Autodesk Fusion 360 part; units mm, degrees
(part 4 of 5)
  spline S979 degree 3 poles (-60.6177, -130.3554) (-60.6177, -130.0705) (-60.5544, -129.9545) (-60.3222, -129.8384) knots 0 0 0 0 1 1 1 1
  spline S980 degree 3 poles (-60.3222, -129.8384) (-60.1639, -129.754) (-60.0268, -129.6801) (-60.0162, -129.6695) knots 0 0 0 0 1 1 1 1
  spline S981 degree 2 poles (-60.0162, -129.6695) (-60.0795, -129.8911) (-60.1639, -130.1655) knots 0 0 0 1 1 1
  spline S982 degree 3 poles (-57.3993, -130.2816) (-56.819, -130.5665) (-56.1331, -130.9463) (-55.8798, -131.1152) knots 0 0 0 0 1 1 1 1
  line L170 (-55.8798, -131.1152) -> (-55.405, -131.4423)
  line L171 (-55.405, -131.4423) -> (-54.7508, -131.0308)
  spline S983 degree 3 poles (-54.7508, -131.0308) (-53.9805, -130.5665) (-53.0097, -130.06) (-52.9675, -130.1127) knots 0 0 0 0 1 1 1 1
  spline S984 degree 3 poles (-52.9675, -130.1127) (-52.9464, -130.1338) (-52.883, -130.5137) (-52.8197, -130.9674) knots 0 0 0 0 1 1 1 1
  spline S985 degree 3 poles (-52.8197, -130.9674) (-52.6931, -131.8855) (-52.672, -132.8985) (-52.767, -133.4894) knots 0 0 0 0 1 1 1 1
  line L172 (-52.767, -133.4894) -> (-52.8408, -133.8904)
  line L173 (-52.8408, -133.8904) -> (-53.379, -133.8904)
  spline S986 degree 3 poles (-53.379, -133.8904) (-53.9805, -133.8904) (-55.3733, -133.5527) (-55.616, -133.3522) knots 0 0 0 0 1 1 1 1
  spline S987 degree 3 poles (-55.616, -133.3522) (-55.9009, -133.1201) (-55.8693, -133.3206) (-55.5527, -133.6899) knots 0 0 0 0 1 1 1 1
  spline S988 degree 3 poles (-55.5527, -133.6899) (-55.3839, -133.8904) (-55.2467, -133.9959) (-55.2361, -133.9326) knots 0 0 0 0 1 1 1 1
  spline S989 degree 3 poles (-55.2361, -133.9326) (-55.2361, -133.8798) (-55.2995, -133.7637) (-55.3628, -133.6899) knots 0 0 0 0 1 1 1 1
  spline S990 degree 3 poles (-55.3628, -133.6899) (-55.4683, -133.5738) (-55.4683, -133.5632) (-55.3733, -133.616) knots 0 0 0 0 1 1 1 1
  spline S991 degree 3 poles (-55.3733, -133.616) (-55.2995, -133.6582) (-55.1517, -133.711) (-55.0568, -133.7321) knots 0 0 0 0 1 1 1 1
  spline S992 degree 3 poles (-55.0568, -133.7321) (-54.9512, -133.7532) (-54.5081, -133.8482) (-54.0754, -133.9431) knots 0 0 0 0 1 1 1 1
  spline S993 degree 3 poles (-54.0754, -133.9431) (-53.6428, -134.0381) (-53.2102, -134.1225) (-53.1152, -134.1331) knots 0 0 0 0 1 1 1 1
  spline S994 degree 3 poles (-53.1152, -134.1331) (-52.9675, -134.1436) (-52.9569, -134.1858) (-53.0835, -134.4918) knots 0 0 0 0 1 1 1 1
  spline S995 degree 3 poles (-53.0835, -134.4918) (-53.1679, -134.6818) (-53.2313, -134.9456) (-53.2313, -135.0827) knots 0 0 0 0 1 1 1 1
  spline S996 degree 3 poles (-53.2313, -135.0827) (-53.2313, -135.5576) (-53.3579, -135.5787) (-56.1225, -135.5681) knots 0 0 0 0 1 1 1 1
  spline S997 degree 3 poles (-56.1225, -135.5681) (-59.0243, -135.547) (-58.866, -135.5892) (-58.9188, -134.7978) knots 0 0 0 0 1 1 1 1
  spline S998 degree 3 poles (-58.9188, -134.7978) (-58.9399, -134.5657) (-59.0243, -134.2702) (-59.1087, -134.1331) knots 0 0 0 0 1 1 1 1
  spline S999 degree 3 poles (-59.1087, -134.1331) (-59.2565, -133.9115) (-59.2565, -133.8904) (-59.0771, -133.8904) knots 0 0 0 0 1 1 1 1
  spline S1000 degree 3 poles (-59.0771, -133.8904) (-58.961, -133.8904) (-58.6339, -133.9642) (-58.349, -134.0486) knots 0 0 0 0 1 1 1 1
  spline S1001 degree 3 poles (-58.349, -134.0486) (-57.8214, -134.2069) (-56.7451, -134.1858) (-56.2386, -133.9959) knots 0 0 0 0 1 1 1 1
  spline S1002 degree 3 poles (-56.2386, -133.9959) (-56.1225, -133.9537) (-55.8693, -133.9853) (-55.6582, -134.0697) knots 0 0 0 0 1 1 1 1
  line L174 (-55.6582, -134.0697) -> (-55.2889, -134.2175)
  line L175 (-55.2889, -134.2175) -> (-55.5527, -133.9959)
  spline S1003 degree 3 poles (-55.5527, -133.9959) (-55.7532, -133.8376) (-55.9009, -133.7954) (-56.1331, -133.8482) knots 0 0 0 0 1 1 1 1
  spline S1004 degree 3 poles (-56.1331, -133.8482) (-57.2621, -134.1014) (-58.6339, -134.0064) (-59.2143, -133.6266) knots 0 0 0 0 1 1 1 1
  spline S1005 degree 3 poles (-59.2143, -133.6266) (-59.6469, -133.3417) (-59.6469, -131.4845) (-59.2248, -130.0916) knots 0 0 0 0 1 1 1 1
  spline S1006 degree 3 poles (-59.2248, -130.0916) (-59.0982, -129.6801) (-59.0665, -129.659) (-58.7711, -129.7118) knots 0 0 0 0 1 1 1 1
  spline S1007 degree 3 poles (-58.7711, -129.7118) (-58.5917, -129.7434) (-57.9797, -130.0072) (-57.3993, -130.2816) knots 0 0 0 0 1 1 1 1
  spline S1008 degree 3 poles (-42.0883, -129.7434) (-42.1938, -129.8489) (-42.5737, -129.8595) (-42.5104, -129.754) knots 0 0 0 0 1 1 1 1
  spline S1009 degree 3 poles (-42.5104, -129.754) (-42.4787, -129.7118) (-42.3521, -129.6695) (-42.236, -129.6695) knots 0 0 0 0 1 1 1 1
  spline S1010 degree 3 poles (-42.236, -129.6695) (-42.1094, -129.6695) (-42.0461, -129.7012) (-42.0883, -129.7434) knots 0 0 0 0 1 1 1 1
  spline S1011 degree 3 poles (-48.7678, -132.3076) (-48.7572, -132.6241) (-48.7889, -132.9829) (-48.8205, -133.099) knots 0 0 0 0 1 1 1 1
  spline S1012 degree 3 poles (-48.8205, -133.099) (-48.9577, -133.5527) (-49.1054, -133.8693) (-49.2004, -133.9326) knots 0 0 0 0 1 1 1 1
  spline S1013 degree 3 poles (-49.2004, -133.9326) (-49.3587, -134.0275) (-49.2215, -133.5527) (-49.021, -133.3206) knots 0 0 0 0 1 1 1 1
  spline S1014 degree 3 poles (-49.021, -133.3206) (-48.8627, -133.1306) (-48.8627, -133.1201) (-49.0527, -133.1939) knots 0 0 0 0 1 1 1 1
  spline S1015 degree 3 poles (-49.0527, -133.1939) (-49.232, -133.2572) (-49.2426, -133.2256) (-49.1687, -132.8668) knots 0 0 0 0 1 1 1 1
  spline S1016 degree 3 poles (-49.1687, -132.8668) (-49.1371, -132.6452) (-49.0949, -132.3814) (-49.1054, -132.2759) knots 0 0 0 0 1 1 1 1
  spline S1017 degree 3 poles (-49.1054, -132.2759) (-49.1054, -132.1809) (-49.0632, -132.1176) (-49.021, -132.1493) knots 0 0 0 0 1 1 1 1
  spline S1018 degree 3 poles (-49.021, -132.1493) (-48.9682, -132.1704) (-48.9682, -131.991) (-49.021, -131.7483) knots 0 0 0 0 1 1 1 1
  spline S1019 degree 3 poles (-49.021, -131.7483) (-49.1476, -131.0835) (-49.116, -130.9463) (-48.9366, -131.3579) knots 0 0 0 0 1 1 1 1
  spline S1020 degree 3 poles (-48.9366, -131.3579) (-48.8522, -131.5584) (-48.7678, -131.991) (-48.7678, -132.3076) knots 0 0 0 0 1 1 1 1
  spline S1021 degree 3 poles (-50.2767, -134.1436) (-50.2767, -134.2175) (-50.3611, -134.4707) (-50.4561, -134.6923) knots 0 0 0 0 1 1 1 1
  spline S1022 degree 3 poles (-50.4561, -134.6923) (-50.551, -134.9245) (-50.6249, -135.1672) (-50.6038, -135.2516) knots 0 0 0 0 1 1 1 1
  spline S1023 degree 3 poles (-50.6038, -135.2516) (-50.5721, -135.4099) (-50.8043, -135.5892) (-50.9309, -135.5154) knots 0 0 0 0 1 1 1 1
  spline S1024 degree 3 poles (-50.9309, -135.5154) (-50.9731, -135.4837) (-51.0153, -135.3676) (-51.0153, -135.2516) knots 0 0 0 0 1 1 1 1
  spline S1025 degree 3 poles (-51.0153, -135.2516) (-51.0153, -135.1249) (-50.9731, -135.0722) (-50.8993, -135.1144) knots 0 0 0 0 1 1 1 1
  spline S1026 degree 3 poles (-50.8993, -135.1144) (-50.8148, -135.1672) (-50.8043, -135.1355) (-50.8782, -134.9983) knots 0 0 0 0 1 1 1 1
  spline S1027 degree 3 poles (-50.8782, -134.9983) (-51.0048, -134.7873) (-50.9415, -134.418) (-50.7832, -134.418) knots 0 0 0 0 1 1 1 1
  spline S1028 degree 3 poles (-50.7832, -134.418) (-50.7304, -134.418) (-50.7199, -134.3652) (-50.7621, -134.3019) knots 0 0 0 0 1 1 1 1
  spline S1029 degree 3 poles (-50.7621, -134.3019) (-50.836, -134.1753) (-50.6355, -133.9959) (-50.4033, -133.9959) knots 0 0 0 0 1 1 1 1
  spline S1030 degree 3 poles (-50.4033, -133.9959) (-50.34, -133.9959) (-50.2767, -134.0592) (-50.2767, -134.1436) knots 0 0 0 0 1 1 1 1
  spline S1031 degree 3 poles (-51.7645, -134.418) (-51.8173, -134.5868) (-51.9017, -134.8717) (-51.9545, -135.0405) knots 0 0 0 0 1 1 1 1
  spline S1032 degree 3 poles (-51.9545, -135.0405) (-52.0072, -135.2094) (-52.0178, -135.3887) (-51.9861, -135.431) knots 0 0 0 0 1 1 1 1
  spline S1033 degree 3 poles (-51.9861, -135.431) (-51.9439, -135.4732) (-51.9861, -135.4837) (-52.0705, -135.4521) knots 0 0 0 0 1 1 1 1
  spline S1034 degree 3 poles (-52.0705, -135.4521) (-52.2499, -135.3993) (-52.3238, -134.5235) (-52.1444, -134.5235) knots 0 0 0 0 1 1 1 1
  spline S1035 degree 3 poles (-52.1444, -134.5235) (-52.0811, -134.5235) (-52.0705, -134.4918) (-52.1022, -134.4496) knots 0 0 0 0 1 1 1 1
  spline S1036 degree 3 poles (-52.1022, -134.4496) (-52.1972, -134.3652) (-51.9756, -134.1014) (-51.7962, -134.1014) knots 0 0 0 0 1 1 1 1
  spline S1037 degree 3 poles (-51.7962, -134.1014) (-51.7012, -134.1014) (-51.6907, -134.1753) (-51.7645, -134.418) knots 0 0 0 0 1 1 1 1
  spline S1038 degree 3 poles (-53.2313, -111.3723) (-53.2313, -111.4462) (-53.1363, -111.6045) (-53.0097, -111.7417) knots 0 0 0 0 1 1 1 1
  spline S1039 degree 3 poles (-53.0097, -111.7417) (-52.8408, -111.9421) (-52.8197, -111.9527) (-52.9041, -111.7839) knots 0 0 0 0 1 1 1 1
  spline S1040 degree 3 poles (-52.9041, -111.7839) (-53.0835, -111.4251) (-53.2313, -111.2457) (-53.2313, -111.3723) knots 0 0 0 0 1 1 1 1
  spline S1041 degree 3 poles (-60.2378, -111.6889) (-60.3433, -111.8366) (-60.4066, -111.9843) (-60.375, -112.0055) knots 0 0 0 0 1 1 1 1
  spline S1042 degree 3 poles (-60.375, -112.0055) (-60.3539, -112.0371) (-60.2484, -111.9316) (-60.1534, -111.7733) knots 0 0 0 0 1 1 1 1
  spline S1043 degree 3 poles (-60.1534, -111.7733) (-60.0479, -111.6256) (-59.9846, -111.4779) (-60.0162, -111.4567) knots 0 0 0 0 1 1 1 1
  spline S1044 degree 3 poles (-60.0162, -111.4567) (-60.0373, -111.4251) (-60.1428, -111.5306) (-60.2378, -111.6889) knots 0 0 0 0 1 1 1 1
  spline S1045 degree 3 poles (-60.3433, -115.6248) (-60.3961, -115.7092) (-60.185, -115.7409) (-59.6152, -115.7409) knots 0 0 0 0 1 1 1 1
  spline S1046 degree 3 poles (-59.6152, -115.7409) (-59.1721, -115.7409) (-58.7183, -115.7936) (-58.6128, -115.8464) knots 0 0 0 0 1 1 1 1
  spline S1047 degree 3 poles (-58.6128, -115.8464) (-58.4018, -115.9625) (-58.2118, -115.8042) (-58.4123, -115.6881) knots 0 0 0 0 1 1 1 1
  spline S1048 degree 3 poles (-58.4123, -115.6881) (-58.6339, -115.5509) (-60.2695, -115.4982) (-60.3433, -115.6248) knots 0 0 0 0 1 1 1 1
  spline S1049 degree 3 poles (-52.4082, -116.9227) (-52.3554, -116.9755) (-52.2394, -117.0071) (-52.1655, -116.986) knots 0 0 0 0 1 1 1 1
  spline S1050 degree 3 poles (-52.1655, -116.986) (-52.0811, -116.9544) (-52.1338, -116.9121) (-52.271, -116.8699) knots 0 0 0 0 1 1 1 1
  spline S1051 degree 3 poles (-52.271, -116.8699) (-52.4504, -116.8277) (-52.4926, -116.8383) (-52.4082, -116.9227) knots 0 0 0 0 1 1 1 1
  spline S1052 degree 3 poles (-53.1785, -117.2182) (-53.2102, -117.2709) (-53.1996, -117.3237) (-53.1363, -117.3237) knots 0 0 0 0 1 1 1 1
  spline S1053 degree 3 poles (-53.1363, -117.3237) (-53.0835, -117.3237) (-52.9991, -117.2709) (-52.9675, -117.2182) knots 0 0 0 0 1 1 1 1
  spline S1054 degree 3 poles (-52.9675, -117.2182) (-52.9358, -117.1548) (-52.9464, -117.1126) (-53.0097, -117.1126) knots 0 0 0 0 1 1 1 1
  spline S1055 degree 3 poles (-53.0097, -117.1126) (-53.0624, -117.1126) (-53.1468, -117.1548) (-53.1785, -117.2182) knots 0 0 0 0 1 1 1 1
  spline S1056 degree 3 poles (-50.6249, -117.6086) (-50.6671, -117.6402) (-50.551, -117.7669) (-50.3822, -117.8724) knots 0 0 0 0 1 1 1 1
  spline S1057 degree 3 poles (-50.3822, -117.8724) (-49.9707, -118.1151) (-49.8441, -118.1151) (-50.1395, -117.8618) knots 0 0 0 0 1 1 1 1
  spline S1058 degree 3 poles (-50.1395, -117.8618) (-50.2661, -117.7563) (-50.34, -117.6402) (-50.3083, -117.598) knots 0 0 0 0 1 1 1 1
  spline S1059 degree 3 poles (-50.3083, -117.598) (-50.2661, -117.5664) (-50.3083, -117.5347) (-50.4033, -117.5347) knots 0 0 0 0 1 1 1 1
  spline S1060 degree 3 poles (-50.4033, -117.5347) (-50.4877, -117.5347) (-50.5933, -117.5664) (-50.6249, -117.6086) knots 0 0 0 0 1 1 1 1
  spline S1061 degree 3 poles (-61.8839, -117.9568) (-62.0105, -118.0412) (-62.0105, -118.0623) (-61.8312, -118.0623) knots 0 0 0 0 1 1 1 1
  spline S1062 degree 3 poles (-61.8312, -118.0623) (-61.7151, -118.0623) (-61.5463, -118.0096) (-61.4618, -117.9568) knots 0 0 0 0 1 1 1 1
  spline S1063 degree 3 poles (-61.4618, -117.9568) (-61.3352, -117.8724) (-61.3352, -117.8513) (-61.5146, -117.8513) knots 0 0 0 0 1 1 1 1
  spline S1064 degree 3 poles (-61.5146, -117.8513) (-61.6307, -117.8513) (-61.7995, -117.904) (-61.8839, -117.9568) knots 0 0 0 0 1 1 1 1
  spline S1065 degree 3 poles (-61.2086, -118.0307) (-61.1769, -118.094) (-61.2297, -118.1784) (-61.3141, -118.21) knots 0 0 0 0 1 1 1 1
  spline S1066 degree 3 poles (-61.3141, -118.21) (-61.3985, -118.2417) (-61.4618, -118.3261) (-61.4618, -118.3894) knots 0 0 0 0 1 1 1 1
  spline S1067 degree 3 poles (-61.4618, -118.3894) (-61.4618, -118.4633) (-61.3563, -118.4211) (-61.2191, -118.2945) knots 0 0 0 0 1 1 1 1
  spline S1068 degree 3 poles (-61.2191, -118.2945) (-61.082, -118.1678) (-60.8393, -118.0518) (-60.6599, -118.0518) knots 0 0 0 0 1 1 1 1
  spline S1069 degree 3 poles (-60.6599, -118.0518) (-60.4911, -118.0412) (-60.2062, -117.999) (-60.0373, -117.9568) knots 0 0 0 0 1 1 1 1
  spline S1070 degree 3 poles (-60.0373, -117.9568) (-59.8157, -117.904) (-59.9529, -117.8829) (-60.4805, -117.8935) knots 0 0 0 0 1 1 1 1
  spline S1071 degree 3 poles (-60.4805, -117.8935) (-61.0187, -117.904) (-61.2403, -117.9462) (-61.2086, -118.0307) knots 0 0 0 0 1 1 1 1
  spline S1072 degree 3 poles (-51.965, -118.8748) (-52.1022, -119.2652) (-52.2288, -119.6662) (-52.2605, -119.7506) knots 0 0 0 0 1 1 1 1
  spline S1073 degree 3 poles (-52.2605, -119.7506) (-52.2921, -119.8562) (-52.2816, -119.8773) (-52.1972, -119.8034) knots 0 0 0 0 1 1 1 1
  spline S1074 degree 3 poles (-52.1972, -119.8034) (-52.0811, -119.6873) (-51.6274, -118.2523) (-51.6907, -118.1889) knots 0 0 0 0 1 1 1 1
  spline S1075 degree 3 poles (-51.6907, -118.1889) (-51.7118, -118.1678) (-51.8384, -118.4738) (-51.965, -118.8748) knots 0 0 0 0 1 1 1 1
  spline S1076 degree 3 poles (-51.0681, -118.8537) (-51.1631, -119.1914) (-51.2158, -119.4763) (-51.1947, -119.5079) knots 0 0 0 0 1 1 1 1
  spline S1077 degree 3 poles (-51.1947, -119.5079) (-51.1631, -119.529) (-51.0575, -119.2864) (-50.9626, -118.9592) knots 0 0 0 0 1 1 1 1
  spline S1078 degree 3 poles (-50.9626, -118.9592) (-50.8676, -118.6216) (-50.8148, -118.3367) (-50.836, -118.305) knots 0 0 0 0 1 1 1 1
  spline S1079 degree 3 poles (-50.836, -118.305) (-50.8676, -118.2839) (-50.9731, -118.5266) (-51.0681, -118.8537) knots 0 0 0 0 1 1 1 1
  spline S1080 degree 3 poles (-52.7037, -118.3894) (-52.7037, -118.4105) (-52.7986, -118.6954) (-52.9147, -119.0014) knots 0 0 0 0 1 1 1 1
  spline S1081 degree 3 poles (-52.9147, -119.0014) (-53.0308, -119.318) (-53.1046, -119.6029) (-53.073, -119.624) knots 0 0 0 0 1 1 1 1
  spline S1082 degree 3 poles (-53.073, -119.624) (-53.0519, -119.6557) (-52.978, -119.5396) (-52.9147, -119.3708) knots 0 0 0 0 1 1 1 1
  spline S1083 degree 3 poles (-52.9147, -119.3708) (-52.8514, -119.2019) (-52.7459, -118.9276) (-52.6826, -118.7693) knots 0 0 0 0 1 1 1 1
  spline S1084 degree 3 poles (-52.6826, -118.7693) (-52.6192, -118.611) (-52.5981, -118.4527) (-52.6403, -118.4105) knots 0 0 0 0 1 1 1 1
  spline S1085 degree 3 poles (-52.6403, -118.4105) (-52.672, -118.3789) (-52.7037, -118.3683) (-52.7037, -118.3894) knots 0 0 0 0 1 1 1 1
  spline S1086 degree 3 poles (-60.1112, -119.4341) (-60.2589, -119.8984) (-60.3539, -120.2782) (-60.3117, -120.2782) knots 0 0 0 0 1 1 1 1
  spline S1087 degree 3 poles (-60.3117, -120.2782) (-60.2378, -120.2782) (-59.7419, -118.6954) (-59.8052, -118.6321) knots 0 0 0 0 1 1 1 1
  spline S1088 degree 3 poles (-59.8052, -118.6321) (-59.8157, -118.611) (-59.9635, -118.9803) (-60.1112, -119.4341) knots 0 0 0 0 1 1 1 1
  spline S1089 degree 3 poles (-59.1404, -119.1281) (-59.2037, -119.3813) (-59.2987, -119.6979) (-59.3514, -119.8245) knots 0 0 0 0 1 1 1 1
  spline S1090 degree 3 poles (-59.3514, -119.8245) (-59.4042, -119.9617) (-59.4148, -120.0672) (-59.362, -120.0672) knots 0 0 0 0 1 1 1 1
  spline S1091 degree 3 poles (-59.362, -120.0672) (-59.267, -120.0672) (-58.8977, -118.801) (-58.9716, -118.7271) knots 0 0 0 0 1 1 1 1
  spline S1092 degree 3 poles (-58.9716, -118.7271) (-59.0032, -118.6954) (-59.0771, -118.8854) (-59.1404, -119.1281) knots 0 0 0 0 1 1 1 1
  spline S1093 degree 3 poles (-61.0081, -119.4341) (-61.1242, -119.7823) (-61.198, -120.0672) (-61.1558, -120.0672) knots 0 0 0 0 1 1 1 1
  spline S1094 degree 3 poles (-61.1558, -120.0672) (-61.1242, -120.0672) (-60.9976, -119.7823) (-60.8709, -119.4341) knots 0 0 0 0 1 1 1 1
  spline S1095 degree 3 poles (-60.8709, -119.4341) (-60.7443, -119.0859) (-60.681, -118.801) (-60.7232, -118.801) knots 0 0 0 0 1 1 1 1
  spline S1096 degree 3 poles (-60.7232, -118.801) (-60.7549, -118.801) (-60.8815, -119.0859) (-61.0081, -119.4341) knots 0 0 0 0 1 1 1 1
  spline S1097 degree 3 poles (-56.228, -120.0566) (-56.9561, -120.1094) (-57.0828, -120.1516) (-57.2621, -120.3838) knots 0 0 0 0 1 1 1 1
  spline S1098 degree 3 poles (-57.2621, -120.3838) (-57.3677, -120.5315) (-57.4837, -120.8269) (-57.5154, -121.0274) knots 0 0 0 0 1 1 1 1
  spline S1099 degree 3 poles (-57.5154, -121.0274) (-57.5681, -121.344) (-57.5365, -121.4495) (-57.336, -121.6395) knots 0 0 0 0 1 1 1 1
  spline S1100 degree 3 poles (-57.336, -121.6395) (-57.1144, -121.8505) (-57.0089, -121.8716) (-56.5024, -121.8083) knots 0 0 0 0 1 1 1 1
  spline S1101 degree 3 poles (-56.5024, -121.8083) (-56.1858, -121.7661) (-55.9009, -121.7133) (-55.8798, -121.6922) knots 0 0 0 0 1 1 1 1
  spline S1102 degree 3 poles (-55.8798, -121.6922) (-55.7637, -121.5867) (-55.9642, -121.5656) (-56.3969, -121.65) knots 0 0 0 0 1 1 1 1
  spline S1103 degree 3 poles (-56.3969, -121.65) (-56.9139, -121.745) (-57.1777, -121.6606) (-57.3466, -121.3334) knots 0 0 0 0 1 1 1 1
  spline S1104 degree 3 poles (-57.3466, -121.3334) (-57.4943, -121.0591) (-57.2938, -120.4998) (-57.1144, -120.6792) knots 0 0 0 0 1 1 1 1
  spline S1105 degree 3 poles (-57.1144, -120.6792) (-56.935, -120.8586) (-56.8506, -120.8375) (-56.7873, -120.6054) knots 0 0 0 0 1 1 1 1
  spline S1106 degree 3 poles (-56.7873, -120.6054) (-56.7451, -120.4471) (-56.5974, -120.4049) (-55.9115, -120.3521) knots 0 0 0 0 1 1 1 1
  spline S1107 degree 3 poles (-55.9115, -120.3521) (-55.1834, -120.2993) (-55.0568, -120.3205) (-54.909, -120.4893) knots 0 0 0 0 1 1 1 1
  spline S1108 degree 3 poles (-54.909, -120.4893) (-54.7824, -120.637) (-54.7085, -120.6581) (-54.6136, -120.5631) knots 0 0 0 0 1 1 1 1
  spline S1109 degree 3 poles (-54.6136, -120.5631) (-54.3603, -120.3099) (-54.1809, -120.943) (-54.392, -121.344) knots 0 0 0 0 1 1 1 1
  spline S1110 degree 3 poles (-54.392, -121.344) (-54.487, -121.5023) (-54.6241, -121.5445) (-55.1623, -121.555) knots 0 0 0 0 1 1 1 1
  line L176 (-55.1623, -121.555) -> (-55.8165, -121.5656)
  line L177 (-55.8165, -121.5656) -> (-55.2573, -121.6606)
  spline S1111 degree 3 poles (-55.2573, -121.6606) (-54.5925, -121.7766) (-54.3498, -121.6817) (-54.202, -121.2385) knots 0 0 0 0 1 1 1 1
  spline S1112 degree 3 poles (-54.202, -121.2385) (-54.0121, -120.7003) (-54.5608, -119.9406) (-55.1201, -119.9828) knots 0 0 0 0 1 1 1 1
  spline S1113 degree 3 poles (-55.1201, -119.9828) (-55.2678, -119.9933) (-55.7743, -120.025) (-56.228, -120.0566) knots 0 0 0 0 1 1 1 1
  spline S1114 degree 3 poles (-54.7085, -120.2255) (-54.6347, -120.3205) (-54.603, -120.4154) (-54.6452, -120.4576) knots 0 0 0 0 1 1 1 1
  spline S1115 degree 3 poles (-54.6452, -120.4576) (-54.6769, -120.4998) (-54.7719, -120.4471) (-54.8457, -120.3627) knots 0 0 0 0 1 1 1 1
  spline S1116 degree 3 poles (-54.8457, -120.3627) (-54.909, -120.2677) (-55.0673, -120.1727) (-55.1834, -120.1411) knots 0 0 0 0 1 1 1 1
  spline S1117 degree 3 poles (-55.1834, -120.1411) (-55.3522, -120.0989) (-55.3311, -120.0883) (-55.1201, -120.0778) knots 0 0 0 0 1 1 1 1
  spline S1118 degree 3 poles (-55.1201, -120.0778) (-54.9618, -120.0778) (-54.7824, -120.1411) (-54.7085, -120.2255) knots 0 0 0 0 1 1 1 1
  spline S1119 degree 3 poles (-56.1225, -120.2677) (-56.7134, -120.3205) (-56.8612, -120.3732) (-56.9245, -120.5315) knots 0 0 0 0 1 1 1 1
  spline S1120 degree 3 poles (-56.9245, -120.5315) (-56.9772, -120.6792) (-57.0194, -120.7003) (-57.0722, -120.6054) knots 0 0 0 0 1 1 1 1
  spline S1121 degree 3 poles (-57.0722, -120.6054) (-57.2516, -120.3205) (-56.9139, -120.1727) (-56.1436, -120.1938) knots 0 0 0 0 1 1 1 1
  line L178 (-56.1436, -120.1938) -> (-55.3944, -120.2149)
  line L179 (-55.3944, -120.2149) -> (-56.1225, -120.2677)
  spline S1122 degree 3 poles (-52.9675, -115.3082) (-52.767, -115.4032) (-52.767, -115.4138) (-52.9886, -115.4138) knots 0 0 0 0 1 1 1 1
  spline S1123 degree 3 poles (-52.9886, -115.4138) (-53.3051, -115.4243) (-53.5478, -115.5298) (-53.5478, -115.6565) knots 0 0 0 0 1 1 1 1
  spline S1124 degree 3 poles (-53.5478, -115.6565) (-53.5478, -115.7198) (-53.474, -115.7303) (-53.3579, -115.6881) knots 0 0 0 0 1 1 1 1
  spline S1125 degree 3 poles (-53.3579, -115.6881) (-53.2629, -115.6353) (-52.8197, -115.5509) (-52.3871, -115.4771) knots 0 0 0 0 1 1 1 1
  spline S1126 degree 3 poles (-52.3871, -115.4771) (-51.6168, -115.3504) (-51.6062, -115.3399) (-52.1233, -115.3293) knots 0 0 0 0 1 1 1 1
  spline S1127 degree 3 poles (-52.1233, -115.3293) (-52.4082, -115.3188) (-52.767, -115.2871) (-52.9147, -115.266) knots 0 0 0 0 1 1 1 1
  spline S1128 degree 3 poles (-52.9147, -115.266) (-53.1468, -115.2133) (-53.1468, -115.2238) (-52.9675, -115.3082) knots 0 0 0 0 1 1 1 1
  spline S1129 degree 3 poles (-51.5429, -117.2709) (-51.5429, -117.292) (-51.448, -117.3659) (-51.3319, -117.4292) knots 0 0 0 0 1 1 1 1
  spline S1130 degree 3 poles (-51.3319, -117.4292) (-51.1631, -117.5242) (-51.142, -117.5136) (-51.1842, -117.3764) knots 0 0 0 0 1 1 1 1
  spline S1131 degree 3 poles (-51.1842, -117.3764) (-51.2369, -117.2393) (-51.5429, -117.1443) (-51.5429, -117.2709) knots 0 0 0 0 1 1 1 1
  spline S1132 degree 3 poles (-59.5097, -117.1126) (-59.4781, -117.1654) (-59.3936, -117.2182) (-59.3409, -117.2182) knots 0 0 0 0 1 1 1 1
  spline S1133 degree 3 poles (-59.3409, -117.2182) (-59.2776, -117.2182) (-59.267, -117.1654) (-59.2987, -117.1126) knots 0 0 0 0 1 1 1 1
  spline S1134 degree 3 poles (-59.2987, -117.1126) (-59.3303, -117.0493) (-59.4148, -117.0071) (-59.4675, -117.0071) knots 0 0 0 0 1 1 1 1
  spline S1135 degree 3 poles (-59.4675, -117.0071) (-59.5308, -117.0071) (-59.5414, -117.0493) (-59.5097, -117.1126) knots 0 0 0 0 1 1 1 1
  spline S1136 degree 3 poles (-54.3392, -126.5039) (-54.2232, -126.5567) (-54.0543, -126.5989) (-53.9699, -126.5989) knots 0 0 0 0 1 1 1 1
  spline S1137 degree 3 poles (-53.9699, -126.5989) (-53.8749, -126.5989) (-53.8855, -126.5567) (-54.0227, -126.5039) knots 0 0 0 0 1 1 1 1
  spline S1138 degree 3 poles (-54.0227, -126.5039) (-54.1387, -126.4512) (-54.3076, -126.409) (-54.392, -126.409) knots 0 0 0 0 1 1 1 1
  spline S1139 degree 3 poles (-54.392, -126.409) (-54.487, -126.409) (-54.4764, -126.4512) (-54.3392, -126.5039) knots 0 0 0 0 1 1 1 1
  spline S1140 degree 3 poles (-52.5454, -126.2401) (-53.5162, -127.1054) (-54.4131, -127.4536) (-55.6688, -127.4642) knots 0 0 0 0 1 1 1 1
  spline S1141 degree 3 poles (-55.6688, -127.4642) (-56.6501, -127.4747) (-57.1461, -127.3481) (-57.8003, -126.926) knots 0 0 0 0 1 1 1 1
  spline S1142 degree 3 poles (-57.8003, -126.926) (-58.349, -126.5884) (-58.4545, -126.5461) (-58.3384, -126.7361) knots 0 0 0 0 1 1 1 1
  spline S1143 degree 3 poles (-58.3384, -126.7361) (-58.2962, -126.8099) (-58.3068, -126.8205) (-58.3912, -126.7783) knots 0 0 0 0 1 1 1 1
  spline S1144 degree 3 poles (-58.3912, -126.7783) (-58.4545, -126.7361) (-58.4862, -126.6622) (-58.4651, -126.62) knots 0 0 0 0 1 1 1 1
  spline S1145 degree 3 poles (-58.4651, -126.62) (-58.3807, -126.4934) (-59.0032, -125.9447) (-59.1404, -126.0291) knots 0 0 0 0 1 1 1 1
  spline S1146 degree 3 poles (-59.1404, -126.0291) (-59.2248, -126.0819) (-59.2248, -126.1346) (-59.1298, -126.2507) knots 0 0 0 0 1 1 1 1
  spline S1147 degree 3 poles (-59.1298, -126.2507) (-59.0665, -126.3246) (-58.961, -126.3668) (-58.8977, -126.3246) knots 0 0 0 0 1 1 1 1
  spline S1148 degree 3 poles (-58.8977, -126.3246) (-58.8449, -126.2929) (-58.8238, -126.314) (-58.866, -126.3773) knots 0 0 0 0 1 1 1 1
  spline S1149 degree 3 poles (-58.866, -126.3773) (-58.961, -126.5356) (-58.138, -127.1793) (-57.3888, -127.5275) knots 0 0 0 0 1 1 1 1
  spline S1150 degree 3 poles (-57.3888, -127.5275) (-56.8506, -127.7807) (-56.629, -127.8229) (-55.8165, -127.8124) knots 0 0 0 0 1 1 1 1
  spline S1151 degree 3 poles (-55.8165, -127.8124) (-54.909, -127.8124) (-54.2232, -127.7385) (-54.1071, -127.6225) knots 0 0 0 0 1 1 1 1
  spline S1152 degree 3 poles (-54.1071, -127.6225) (-54.0754, -127.6014) (-54.3076, -127.5908) (-54.6136, -127.6225) knots 0 0 0 0 1 1 1 1
  line L180 (-54.6136, -127.6225) -> (-55.1834, -127.6647)
  line L181 (-55.1834, -127.6647) -> (-54.3603, -127.422)
  spline S1153 degree 3 poles (-54.3603, -127.422) (-53.9066, -127.2742) (-53.4845, -127.116) (-53.4106, -127.0421) knots 0 0 0 0 1 1 1 1
  spline S1154 degree 3 poles (-53.4106, -127.0421) (-53.2418, -126.8733) (-53.073, -126.8944) (-53.2207, -127.0737) knots 0 0 0 0 1 1 1 1
  spline S1155 degree 3 poles (-53.2207, -127.0737) (-53.284, -127.1582) (-53.4845, -127.2742) (-53.6639, -127.3481) knots 0 0 0 0 1 1 1 1
  spline S1156 degree 3 poles (-53.6639, -127.3481) (-53.8327, -127.422) (-53.9488, -127.5064) (-53.9277, -127.538) knots 0 0 0 0 1 1 1 1
  spline S1157 degree 3 poles (-53.9277, -127.538) (-53.8222, -127.6436) (-52.9464, -127.0315) (-52.3871, -126.4617) knots 0 0 0 0 1 1 1 1
  spline S1158 degree 3 poles (-52.3871, -126.4617) (-51.754, -125.8075) (-51.87, -125.6492) (-52.5454, -126.2401) knots 0 0 0 0 1 1 1 1
  spline S1159 degree 3 poles (-52.4926, -126.4512) (-52.7459, -126.715) (-53.0097, -126.926) (-53.0624, -126.926) knots 0 0 0 0 1 1 1 1
  spline S1160 degree 3 poles (-53.0624, -126.926) (-53.1679, -126.926) (-52.1866, -125.9869) (-52.0705, -125.9763) knots 0 0 0 0 1 1 1 1
  spline S1161 degree 3 poles (-52.0705, -125.9763) (-52.0494, -125.9763) (-52.2394, -126.1874) (-52.4926, -126.4512) knots 0 0 0 0 1 1 1 1
  spline S1162 degree 3 poles (-57.9691, -126.9999) (-57.8319, -127.1582) (-57.8425, -127.1582) (-58.0535, -127.0421) knots 0 0 0 0 1 1 1 1
  spline S1163 degree 3 poles (-58.0535, -127.0421) (-58.3068, -126.9155) (-58.3595, -126.8205) (-58.2013, -126.8205) knots 0 0 0 0 1 1 1 1
  spline S1164 degree 3 poles (-58.2013, -126.8205) (-58.1485, -126.8205) (-58.043, -126.8944) (-57.9691, -126.9999) knots 0 0 0 0 1 1 1 1
  spline S1165 degree 3 poles (-57.0405, -127.4642) (-56.8612, -127.5169) (-56.8295, -127.5486) (-56.9561, -127.5486) knots 0 0 0 0 1 1 1 1
  spline S1166 degree 3 poles (-56.9561, -127.5486) (-57.1461, -127.5591) (-57.7686, -127.2848) (-57.7686, -127.1793) knots 0 0 0 0 1 1 1 1
  spline S1167 degree 3 poles (-57.7686, -127.1793) (-57.7686, -127.1582) (-57.6631, -127.1898) (-57.5365, -127.2531) knots 0 0 0 0 1 1 1 1
  spline S1168 degree 3 poles (-57.5365, -127.2531) (-57.4099, -127.3164) (-57.1883, -127.4114) (-57.0405, -127.4642) knots 0 0 0 0 1 1 1 1
  spline S1169 degree 3 poles (-55.2573, -127.7174) (-55.1623, -127.8018) (-56.323, -127.7596) (-56.5552, -127.6647) knots 0 0 0 0 1 1 1 1
  spline S1170 degree 3 poles (-56.5552, -127.6647) (-56.6818, -127.6119) (-56.4918, -127.5908) (-56.0381, -127.6225) knots 0 0 0 0 1 1 1 1
  spline S1171 degree 3 poles (-56.0381, -127.6225) (-55.6371, -127.6436) (-55.2889, -127.6858) (-55.2573, -127.7174) knots 0 0 0 0 1 1 1 1
  spline S1172 degree 3 poles (-52.883, -127.5064) (-52.883, -127.5908) (-52.8408, -127.6647) (-52.7881, -127.6647) knots 0 0 0 0 1 1 1 1
  spline S1173 degree 3 poles (-52.7881, -127.6647) (-52.7459, -127.6647) (-52.7037, -127.6225) (-52.7037, -127.5697) knots 0 0 0 0 1 1 1 1
  spline S1174 degree 3 poles (-52.7037, -127.5697) (-52.7037, -127.5064) (-52.7459, -127.4431) (-52.7881, -127.4114) knots 0 0 0 0 1 1 1 1
  spline S1175 degree 3 poles (-52.7881, -127.4114) (-52.8408, -127.3798) (-52.883, -127.422) (-52.883, -127.5064) knots 0 0 0 0 1 1 1 1
  spline S1176 degree 3 poles (-52.5981, -128.0234) (-52.5981, -128.1078) (-52.5243, -128.1923) (-52.4399, -128.2345) knots 0 0 0 0 1 1 1 1
  spline S1177 degree 3 poles (-52.4399, -128.2345) (-52.3027, -128.2767) (-52.2921, -128.2556) (-52.3871, -128.0867) knots 0 0 0 0 1 1 1 1
  spline S1178 degree 3 poles (-52.3871, -128.0867) (-52.5243, -127.844) (-52.5981, -127.8124) (-52.5981, -128.0234) knots 0 0 0 0 1 1 1 1
  spline S1179 degree 3 poles (-50.5933, -127.6647) (-50.5933, -127.7174) (-50.5405, -127.7702) (-50.4772, -127.7702) knots 0 0 0 0 1 1 1 1
  spline S1180 degree 3 poles (-50.4772, -127.7702) (-50.4244, -127.7702) (-50.4033, -127.7174) (-50.435, -127.6647) knots 0 0 0 0 1 1 1 1
  spline S1181 degree 3 poles (-50.435, -127.6647) (-50.4666, -127.6014) (-50.5194, -127.5591) (-50.551, -127.5591) knots 0 0 0 0 1 1 1 1
  spline S1182 degree 3 poles (-50.551, -127.5591) (-50.5721, -127.5591) (-50.5933, -127.6014) (-50.5933, -127.6647) knots 0 0 0 0 1 1 1 1
  spline S1183 degree 3 poles (-49.7491, -133.5738) (-49.8441, -133.6371) (-49.8546, -133.6793) (-49.7807, -133.6793) knots 0 0 0 0 1 1 1 1
  spline S1184 degree 3 poles (-49.7807, -133.6793) (-49.7174, -133.6793) (-49.6225, -133.6266) (-49.5908, -133.5738) knots 0 0 0 0 1 1 1 1
  spline S1185 degree 3 poles (-49.5908, -133.5738) (-49.5064, -133.4472) (-49.5486, -133.4472) (-49.7491, -133.5738) knots 0 0 0 0 1 1 1 1
  spline S1186 degree 3 poles (-58.4756, -127.633) (-58.5178, -127.7385) (-58.6339, -127.8968) (-58.75, -127.9812) knots 0 0 0 0 1 1 1 1
  spline S1187 degree 3 poles (-58.75, -127.9812) (-58.8555, -128.0762) (-58.9716, -128.34) (-59.0032, -128.6038) knots 0 0 0 0 1 1 1 1
  line L182 (-59.0032, -128.6038) -> (-59.0665, -129.0575)
  line L183 (-59.0665, -129.0575) -> (-58.6233, -128.7726)
  spline S1188 degree 3 poles (-58.6233, -128.7726) (-58.3912, -128.6143) (-58.1907, -128.4139) (-58.1907, -128.3189) knots 0 0 0 0 1 1 1 1
  spline S1189 degree 3 poles (-58.1907, -128.3189) (-58.1907, -128.2345) (-58.1063, -128.1078) (-58.0113, -128.034) knots 0 0 0 0 1 1 1 1
  spline S1190 degree 3 poles (-58.0113, -128.034) (-57.853, -127.9179) (-57.853, -127.8757) (-57.9691, -127.728) knots 0 0 0 0 1 1 1 1
  spline S1191 degree 3 poles (-57.9691, -127.728) (-58.043, -127.633) (-58.1485, -127.5908) (-58.2013, -127.6225) knots 0 0 0 0 1 1 1 1
  spline S1192 degree 3 poles (-58.2013, -127.6225) (-58.349, -127.7069) (-58.2013, -127.8863) (-58.0535, -127.8124) knots 0 0 0 0 1 1 1 1
  spline S1193 degree 3 poles (-58.0535, -127.8124) (-57.9586, -127.7596) (-57.9586, -127.7702) (-58.0535, -127.8757) knots 0 0 0 0 1 1 1 1
  spline S1194 degree 3 poles (-58.0535, -127.8757) (-58.2118, -128.0551) (-58.4334, -127.8968) (-58.3701, -127.6541) knots 0 0 0 0 1 1 1 1
  spline S1195 degree 3 poles (-58.3701, -127.6541) (-58.3068, -127.4009) (-58.3807, -127.3903) (-58.4756, -127.633) knots 0 0 0 0 1 1 1 1
  spline S1196 degree 3 poles (-58.2962, -128.1817) (-58.2962, -128.2978) (-58.444, -128.4983) (-58.6233, -128.6249) knots 0 0 0 0 1 1 1 1
  line L184 (-58.6233, -128.6249) -> (-58.9505, -128.857)
  line L185 (-58.9505, -128.857) -> (-58.8766, -128.4983)
  spline S1197 degree 3 poles (-58.8766, -128.4983) (-58.8344, -128.2978) (-58.7394, -128.1078) (-58.6761, -128.0656) knots 0 0 0 0 1 1 1 1
  spline S1198 degree 3 poles (-58.6761, -128.0656) (-58.4651, -127.9179) (-58.2962, -127.9812) (-58.2962, -128.1817) knots 0 0 0 0 1 1 1 1
  spline S1199 degree 3 poles (-58.6656, -128.2028) (-58.7078, -128.2661) (-58.7183, -128.3294) (-58.6867, -128.3611) knots 0 0 0 0 1 1 1 1
  spline S1200 degree 3 poles (-58.6867, -128.3611) (-58.6656, -128.3928) (-58.6128, -128.34) (-58.5811, -128.245) knots 0 0 0 0 1 1 1 1
  spline S1201 degree 3 poles (-58.5811, -128.245) (-58.5073, -128.0656) (-58.5706, -128.034) (-58.6656, -128.2028) knots 0 0 0 0 1 1 1 1
  spline S1202 degree 3 poles (-57.1988, -128.2556) (-57.2305, -128.3716) (-57.3149, -128.5721) (-57.3888, -128.7199) knots 0 0 0 0 1 1 1 1
  spline S1203 degree 3 poles (-57.3888, -128.7199) (-57.5259, -128.9837) (-57.4943, -129.7751) (-57.3466, -129.7751) knots 0 0 0 0 1 1 1 1
  spline S1204 degree 3 poles (-57.3466, -129.7751) (-57.1988, -129.7751) (-56.7029, -128.9626) (-56.7662, -128.8043) knots 0 0 0 0 1 1 1 1
  spline S1205 degree 3 poles (-56.7662, -128.8043) (-56.7978, -128.7199) (-56.7556, -128.5827) (-56.6607, -128.5088) knots 0 0 0 0 1 1 1 1
  spline S1206 degree 3 poles (-56.6607, -128.5088) (-56.5763, -128.435) (-56.5024, -128.3189) (-56.5024, -128.2556) knots 0 0 0 0 1 1 1 1
  spline S1207 degree 3 poles (-56.5024, -128.2556) (-56.5024, -128.1923) (-56.5552, -128.2239) (-56.6185, -128.3189) knots 0 0 0 0 1 1 1 1
  spline S1208 degree 3 poles (-56.6185, -128.3189) (-56.6712, -128.4244) (-56.819, -128.5088) (-56.9245, -128.5088) knots 0 0 0 0 1 1 1 1
  spline S1209 degree 3 poles (-56.9245, -128.5088) (-57.0511, -128.5088) (-57.1355, -128.435) (-57.1355, -128.3189) knots 0 0 0 0 1 1 1 1
  spline S1210 degree 3 poles (-57.1355, -128.3189) (-57.1355, -128.1712) (-57.1144, -128.1606) (-57.03, -128.2978) knots 0 0 0 0 1 1 1 1
  spline S1211 degree 3 poles (-57.03, -128.2978) (-56.9561, -128.4244) (-56.9139, -128.4244) (-56.819, -128.3189) knots 0 0 0 0 1 1 1 1
  spline S1212 degree 3 poles (-56.819, -128.3189) (-56.7662, -128.2556) (-56.7451, -128.2134) (-56.7767, -128.245) knots 0 0 0 0 1 1 1 1
  spline S1213 degree 3 poles (-56.7767, -128.245) (-56.819, -128.2767) (-56.9139, -128.245) (-56.9878, -128.1817) knots 0 0 0 0 1 1 1 1
  spline S1214 degree 3 poles (-56.9878, -128.1817) (-57.1039, -128.0867) (-57.1461, -128.1078) (-57.1988, -128.2556) knots 0 0 0 0 1 1 1 1
  spline S1215 degree 3 poles (-56.8823, -128.7832) (-56.8506, -128.8676) (-56.9245, -129.0892) (-57.0616, -129.2686) knots 0 0 0 0 1 1 1 1
  line L186 (-57.0616, -129.2686) -> (-57.2938, -129.5851)
  line L187 (-57.2938, -129.5851) -> (-57.3254, -129.1947)
  spline S1216 degree 3 poles (-57.3254, -129.1947) (-57.3466, -128.9415) (-57.3043, -128.7621) (-57.2199, -128.7093) knots 0 0 0 0 1 1 1 1
  spline S1217 degree 3 poles (-57.2199, -128.7093) (-57.0194, -128.5827) (-56.9561, -128.5932) (-56.8823, -128.7832) knots 0 0 0 0 1 1 1 1
  spline S1218 degree 3 poles (-57.2094, -128.8781) (-57.241, -128.9731) (-57.241, -129.0681) (-57.2199, -129.0997) knots 0 0 0 0 1 1 1 1
  spline S1219 degree 3 poles (-57.2199, -129.0997) (-57.1883, -129.1314) (-57.1355, -129.0575) (-57.1039, -128.9309) knots 0 0 0 0 1 1 1 1
  spline S1220 degree 3 poles (-57.1039, -128.9309) (-57.0405, -128.6882) (-57.1144, -128.646) (-57.2094, -128.8781) knots 0 0 0 0 1 1 1 1
  spline S1221 degree 3 poles (-55.8165, -128.4561) (-55.7215, -128.7515) (-55.7215, -128.741) (-55.806, -129.0575) knots 0 0 0 0 1 1 1 1
  spline S1222 degree 3 poles (-55.806, -129.0575) (-55.8904, -129.353) (-55.616, -130.4082) (-55.4577, -130.4082) knots 0 0 0 0 1 1 1 1
  spline S1223 degree 3 poles (-55.4577, -130.4082) (-55.405, -130.4082) (-55.2889, -130.1233) (-55.1939, -129.7645) knots 0 0 0 0 1 1 1 1
  spline S1224 degree 3 poles (-55.1939, -129.7645) (-55.0568, -129.2897) (-55.0357, -129.0892) (-55.1306, -128.9837) knots 0 0 0 0 1 1 1 1
  spline S1225 degree 3 poles (-55.1306, -128.9837) (-55.215, -128.8781) (-55.215, -128.7832) (-55.1412, -128.6249) knots 0 0 0 0 1 1 1 1
  spline S1226 degree 3 poles (-55.1412, -128.6249) (-55.0568, -128.4666) (-55.0568, -128.3928) (-55.1517, -128.34) knots 0 0 0 0 1 1 1 1
  spline S1227 degree 3 poles (-55.1517, -128.34) (-55.2256, -128.2978) (-55.2573, -128.2978) (-55.215, -128.3505) knots 0 0 0 0 1 1 1 1
  spline S1228 degree 3 poles (-55.215, -128.3505) (-55.1728, -128.3928) (-55.1834, -128.4983) (-55.2467, -128.5827) knots 0 0 0 0 1 1 1 1
  spline S1229 degree 3 poles (-55.2467, -128.5827) (-55.3839, -128.741) (-55.6582, -128.7726) (-55.6582, -128.6143) knots 0 0 0 0 1 1 1 1
  spline S1230 degree 3 poles (-55.6582, -128.6143) (-55.6582, -128.5616) (-55.5844, -128.5405) (-55.4999, -128.5721) knots 0 0 0 0 1 1 1 1
  spline S1231 degree 3 poles (-55.4999, -128.5721) (-55.405, -128.6143) (-55.3417, -128.5721) (-55.3417, -128.4666) knots 0 0 0 0 1 1 1 1
  spline S1232 degree 3 poles (-55.3417, -128.4666) (-55.3417, -128.2767) (-55.5105, -128.245) (-55.616, -128.4139) knots 0 0 0 0 1 1 1 1
  spline S1233 degree 3 poles (-55.616, -128.4139) (-55.6582, -128.4983) (-55.711, -128.4877) (-55.7849, -128.3928) knots 0 0 0 0 1 1 1 1
  spline S1234 degree 3 poles (-55.7849, -128.3928) (-55.8587, -128.2872) (-55.8693, -128.3083) (-55.8165, -128.4561) knots 0 0 0 0 1 1 1 1
  spline S1235 degree 3 poles (-55.2784, -129.0153) (-55.1939, -129.1525) (-55.2045, -129.3319) (-55.31, -129.7223) knots 0 0 0 0 1 1 1 1
  line L188 (-55.31, -129.7223) -> (-55.4683, -130.2499)
  line L189 (-55.4683, -130.2499) -> (-55.616, -129.8278)
  spline S1236 degree 3 poles (-55.616, -129.8278) (-55.7954, -129.3108) (-55.7954, -129.1103) (-55.6371, -128.952) knots 0 0 0 0 1 1 1 1
  spline S1237 degree 3 poles (-55.6371, -128.952) (-55.4683, -128.7832) (-55.4155, -128.7937) (-55.2784, -129.0153) knots 0 0 0 0 1 1 1 1
  spline S1238 degree 3 poles (-55.5949, -129.2053) (-55.6266, -129.3002) (-55.616, -129.448) (-55.5527, -129.5429) knots 0 0 0 0 1 1 1 1
  spline S1239 degree 3 poles (-55.5527, -129.5429) (-55.4788, -129.6907) (-55.4577, -129.6484) (-55.4472, -129.3741) knots 0 0 0 0 1 1 1 1
  spline S1240 degree 3 poles (-55.4472, -129.3741) (-55.4472, -129.0048) (-55.4999, -128.9415) (-55.5949, -129.2053) knots 0 0 0 0 1 1 1 1
  spline S1241 degree 3 poles (-54.1598, -128.0762) (-54.1176, -128.2134) (-53.9699, -128.245) (-53.9594, -128.1184) knots 0 0 0 0 1 1 1 1
  spline S1242 degree 3 poles (-53.9594, -128.1184) (-53.9594, -128.0762) (-54.0121, -128.0234) (-54.0754, -127.9918) knots 0 0 0 0 1 1 1 1
  spline S1243 degree 3 poles (-54.0754, -127.9918) (-54.1493, -127.9707) (-54.1915, -128.0129) (-54.1598, -128.0762) knots 0 0 0 0 1 1 1 1
  spline S1244 degree 3 poles (-51.8595, -106.7294) (-51.7962, -106.8983) (-51.5535, -107.2781) (-51.3213, -107.5842) knots 0 0 0 0 1 1 1 1
  spline S1245 degree 3 poles (-51.3213, -107.5842) (-51.0786, -107.8902) (-50.7304, -108.4283) (-50.5299, -108.7976) knots 0 0 0 0 1 1 1 1
  spline S1246 degree 3 poles (-50.5299, -108.7976) (-50.34, -109.167) (-50.1712, -109.4202) (-50.1712, -109.3674) knots 0 0 0 0 1 1 1 1
  spline S1247 degree 3 poles (-50.1712, -109.3674) (-50.1712, -109.1775) (-50.8043, -108.0484) (-51.2158, -107.4997) knots 0 0 0 0 1 1 1 1
  spline S1248 degree 3 poles (-51.2158, -107.4997) (-51.4585, -107.1832) (-51.6485, -106.8772) (-51.6485, -106.8139) knots 0 0 0 0 1 1 1 1
  spline S1249 degree 3 poles (-51.6485, -106.8139) (-51.6485, -106.7505) (-51.7223, -106.6345) (-51.8067, -106.5606) knots 0 0 0 0 1 1 1 1
  spline S1250 degree 3 poles (-51.8067, -106.5606) (-51.9545, -106.4445) (-51.9545, -106.4551) (-51.8595, -106.7294) knots 0 0 0 0 1 1 1 1
  spline S1251 degree 3 poles (-49.327, -107.2148) (-49.3165, -107.4048) (-49.0632, -107.7213) (-48.9155, -107.7213) knots 0 0 0 0 1 1 1 1
  spline S1252 degree 3 poles (-48.9155, -107.7213) (-48.7361, -107.7213) (-48.7783, -107.4575) (-48.9893, -107.2676) knots 0 0 0 0 1 1 1 1
  spline S1253 degree 3 poles (-48.9893, -107.2676) (-49.2215, -107.0565) (-49.327, -107.046) (-49.327, -107.2148) knots 0 0 0 0 1 1 1 1
  spline S1254 degree 3 poles (-49.6225, -107.6264) (-49.6014, -107.7002) (-49.5169, -107.7846) (-49.4431, -107.8057) knots 0 0 0 0 1 1 1 1
  spline S1255 degree 3 poles (-49.4431, -107.8057) (-49.3587, -107.8374) (-49.3165, -107.7952) (-49.3481, -107.7108) knots 0 0 0 0 1 1 1 1
  spline S1256 degree 3 poles (-49.3481, -107.7108) (-49.3692, -107.6369) (-49.4536, -107.5525) (-49.5275, -107.5314) knots 0 0 0 0 1 1 1 1
  spline S1257 degree 3 poles (-49.5275, -107.5314) (-49.6119, -107.4997) (-49.6541, -107.5419) (-49.6225, -107.6264) knots 0 0 0 0 1 1 1 1
  spline S1258 degree 3 poles (-52.8092, -107.9218) (-52.8092, -108.1329) (-52.6298, -108.3122) (-52.5243, -108.2173) knots 0 0 0 0 1 1 1 1
  spline S1259 degree 3 poles (-52.5243, -108.2173) (-52.4504, -108.1329) (-52.5981, -107.7213) (-52.7142, -107.7213) knots 0 0 0 0 1 1 1 1
  spline S1260 degree 3 poles (-52.7142, -107.7213) (-52.767, -107.7213) (-52.8092, -107.8163) (-52.8092, -107.9218) knots 0 0 0 0 1 1 1 1
  spline S1261 degree 3 poles (-52.0072, -108.2384) (-52.1761, -108.5022) (-52.1866, -109.2725) (-52.0283, -109.6207) knots 0 0 0 0 1 1 1 1
  spline S1262 degree 3 poles (-52.0283, -109.6207) (-51.8384, -110.0639) (-51.8173, -109.9795) (-51.9756, -109.3463) knots 0 0 0 0 1 1 1 1
  spline S1263 degree 3 poles (-51.9756, -109.3463) (-52.0705, -108.9876) (-52.0705, -108.8398) (-51.9756, -108.7449) knots 0 0 0 0 1 1 1 1
  spline S1264 degree 3 poles (-51.9756, -108.7449) (-51.8912, -108.6605) (-51.8595, -108.6816) (-51.8595, -108.8504) knots 0 0 0 0 1 1 1 1
  spline S1265 degree 3 poles (-51.8595, -108.8504) (-51.8595, -109.1142) (-51.5324, -110.5915) (-51.4796, -110.5493) knots 0 0 0 0 1 1 1 1
  spline S1266 degree 3 poles (-51.4796, -110.5493) (-51.4374, -110.4965) (-51.8173, -108.2595) (-51.8912, -108.1856) knots 0 0 0 0 1 1 1 1
  spline S1267 degree 3 poles (-51.8912, -108.1856) (-51.9228, -108.154) (-51.9756, -108.1751) (-52.0072, -108.2384) knots 0 0 0 0 1 1 1 1
  spline S1268 degree 3 poles (-62.0211, -108.5866) (-62.7597, -109.5574) (-63.5828, -111.8261) (-63.5617, -112.7757) knots 0 0 0 0 1 1 1 1
  line L190 (-63.5617, -112.7757) -> (-63.5511, -113.2611)
  line L191 (-63.5511, -113.2611) -> (-63.4667, -112.7335)
  spline S1269 degree 3 poles (-63.4667, -112.7335) (-63.2662, -111.4462) (-62.7703, -110.0744) (-62.0633, -108.9032) knots 0 0 0 0 1 1 1 1
  spline S1270 degree 3 poles (-62.0633, -108.9032) (-61.8839, -108.6077) (-61.6729, -108.3544) (-61.599, -108.3544) knots 0 0 0 0 1 1 1 1
  spline S1271 degree 3 poles (-61.599, -108.3544) (-61.3985, -108.3544) (-61.4196, -108.3967) (-61.8839, -109.1986) knots 0 0 0 0 1 1 1 1
  spline S1272 degree 3 poles (-61.8839, -109.1986) (-62.1161, -109.5996) (-62.306, -109.9584) (-62.306, -109.99) knots 0 0 0 0 1 1 1 1
  spline S1273 degree 3 poles (-62.306, -109.99) (-62.306, -110.0322) (-62.3799, -110.2327) (-62.4748, -110.4438) knots 0 0 0 0 1 1 1 1
  spline S1274 degree 3 poles (-62.4748, -110.4438) (-62.7597, -111.098) (-62.8125, -111.2352) (-63.0341, -111.8894) knots 0 0 0 0 1 1 1 1
  spline S1275 degree 3 poles (-63.0341, -111.8894) (-63.1502, -112.2376) (-63.2662, -112.7124) (-63.2979, -112.9446) knots 0 0 0 0 1 1 1 1
  spline S1276 degree 3 poles (-63.2979, -112.9446) (-63.3401, -113.2189) (-63.2662, -113.0607) (-63.0869, -112.5225) knots 0 0 0 0 1 1 1 1
  spline S1277 degree 3 poles (-63.0869, -112.5225) (-62.6859, -111.2668) (-62.1161, -109.8634) (-61.6518, -109.0614) knots 0 0 0 0 1 1 1 1
  spline S1278 degree 3 poles (-61.6518, -109.0614) (-61.4302, -108.6605) (-61.2508, -108.3122) (-61.2508, -108.2911) knots 0 0 0 0 1 1 1 1
  spline S1279 degree 3 poles (-61.2508, -108.2911) (-61.2508, -108.27) (-61.3669, -108.2489) (-61.5041, -108.2489) knots 0 0 0 0 1 1 1 1
  spline S1280 degree 3 poles (-61.5041, -108.2489) (-61.6729, -108.2489) (-61.8523, -108.365) (-62.0211, -108.5866) knots 0 0 0 0 1 1 1 1
  spline S1281 degree 3 poles (-58.8766, -108.576) (-58.9188, -108.7554) (-58.9188, -108.9243) (-58.8871, -108.9559) knots 0 0 0 0 1 1 1 1
  spline S1282 degree 3 poles (-58.8871, -108.9559) (-58.7711, -109.072) (-58.5073, -108.7554) (-58.5073, -108.5022) knots 0 0 0 0 1 1 1 1
  spline S1283 degree 3 poles (-58.5073, -108.5022) (-58.5073, -108.1329) (-58.7922, -108.1856) (-58.8766, -108.576) knots 0 0 0 0 1 1 1 1
  spline S1284 degree 3 poles (-68.3207, -108.4494) (-68.2362, -108.5127) (-68.0991, -108.5655) (-68.0147, -108.5655) knots 0 0 0 0 1 1 1 1
  spline S1285 degree 3 poles (-68.0147, -108.5655) (-67.9408, -108.5655) (-67.582, -108.766) (-67.2233, -108.9981) knots 0 0 0 0 1 1 1 1
  spline S1286 degree 3 poles (-67.2233, -108.9981) (-66.6007, -109.4202) (-66.5901, -109.4308) (-66.8961, -109.0931) knots 0 0 0 0 1 1 1 1
  spline S1287 degree 3 poles (-66.8961, -109.0931) (-67.2655, -108.7027) (-67.6031, -108.5127) (-68.1096, -108.4178) knots 0 0 0 0 1 1 1 1
  spline S1288 degree 3 poles (-68.1096, -108.4178) (-68.384, -108.365) (-68.4367, -108.3756) (-68.3207, -108.4494) knots 0 0 0 0 1 1 1 1
  spline S1289 degree 3 poles (-57.9797, -108.5127) (-57.9797, -108.5971) (-57.9269, -108.671) (-57.8742, -108.671) knots 0 0 0 0 1 1 1 1
  spline S1290 degree 3 poles (-57.8742, -108.671) (-57.8108, -108.671) (-57.7686, -108.5971) (-57.7686, -108.5127) knots 0 0 0 0 1 1 1 1
  spline S1291 degree 3 poles (-57.7686, -108.5127) (-57.7686, -108.4283) (-57.8108, -108.3544) (-57.8742, -108.3544) knots 0 0 0 0 1 1 1 1
  spline S1292 degree 3 poles (-57.8742, -108.3544) (-57.9269, -108.3544) (-57.9797, -108.4283) (-57.9797, -108.5127) knots 0 0 0 0 1 1 1 1
  spline S1293 degree 3 poles (-64.4692, -108.9876) (-64.6486, -109.3252) (-64.6802, -109.6207) (-64.543, -109.6207) knots 0 0 0 0 1 1 1 1
  spline S1294 degree 3 poles (-64.543, -109.6207) (-64.3848, -109.6207) (-64.121, -109.2619) (-64.0471, -108.9559) knots 0 0 0 0 1 1 1 1
  spline S1295 degree 3 poles (-64.0471, -108.9559) (-63.9416, -108.5549) (-64.2476, -108.5655) (-64.4692, -108.9876) knots 0 0 0 0 1 1 1 1
  spline S1296 degree 3 poles (-64.3003, -109.167) (-64.427, -109.378) (-64.4481, -109.3147) (-64.3531, -109.0403) knots 0 0 0 0 1 1 1 1
  spline S1297 degree 3 poles (-64.3531, -109.0403) (-64.3109, -108.9454) (-64.2581, -108.8926) (-64.237, -108.9243) knots 0 0 0 0 1 1 1 1
  spline S1298 degree 3 poles (-64.237, -108.9243) (-64.2054, -108.9454) (-64.237, -109.0614) (-64.3003, -109.167) knots 0 0 0 0 1 1 1 1
  spline S1299 degree 3 poles (-63.7833, -109.3147) (-63.7833, -109.4308) (-63.7305, -109.4941) (-63.6778, -109.4624) knots 0 0 0 0 1 1 1 1
  spline S1300 degree 3 poles (-63.6778, -109.4624) (-63.6145, -109.4308) (-63.5722, -109.3252) (-63.5722, -109.2408) knots 0 0 0 0 1 1 1 1
  spline S1301 degree 3 poles (-63.5722, -109.2408) (-63.5722, -109.1564) (-63.6145, -109.0931) (-63.6778, -109.0931) knots 0 0 0 0 1 1 1 1
  spline S1302 degree 3 poles (-63.6778, -109.0931) (-63.7305, -109.0931) (-63.7833, -109.1881) (-63.7833, -109.3147) knots 0 0 0 0 1 1 1 1
  spline S1303 degree 3 poles (-58.4862, -109.4413) (-58.6445, -109.6312) (-58.7711, -110.7392) (-58.6445, -110.8131) knots 0 0 0 0 1 1 1 1
  spline S1304 degree 3 poles (-58.6445, -110.8131) (-58.5495, -110.8658) (-58.2435, -109.4202) (-58.3279, -109.3358) knots 0 0 0 0 1 1 1 1
  spline S1305 degree 3 poles (-58.3279, -109.3358) (-58.349, -109.3147) (-58.4229, -109.3674) (-58.4862, -109.4413) knots 0 0 0 0 1 1 1 1
  spline S1306 degree 3 poles (-67.371, -109.6207) (-67.371, -109.7473) (-67.1916, -109.7473) (-66.8961, -109.6207) knots 0 0 0 0 1 1 1 1
  spline S1307 degree 3 poles (-66.8961, -109.6207) (-66.7168, -109.5468) (-66.7379, -109.5257) (-67.0228, -109.5257) knots 0 0 0 0 1 1 1 1
  spline S1308 degree 3 poles (-67.0228, -109.5257) (-67.2127, -109.5152) (-67.371, -109.5574) (-67.371, -109.6207) knots 0 0 0 0 1 1 1 1
  spline S1309 degree 3 poles (-66.8434, -110.8236) (-67.2233, -110.8869) (-67.6348, -111.003) (-67.7614, -111.0769) knots 0 0 0 0 1 1 1 1
  spline S1310 degree 3 poles (-67.7614, -111.0769) (-68.0463, -111.2352) (-68.0885, -111.3618) (-67.8142, -111.2246) knots 0 0 0 0 1 1 1 1
  spline S1311 degree 3 poles (-67.8142, -111.2246) (-67.7192, -111.1718) (-67.2866, -111.0663) (-66.8645, -110.9925) knots 0 0 0 0 1 1 1 1
  spline S1312 degree 3 poles (-66.8645, -110.9925) (-66.4424, -110.908) (-66.0731, -110.8131) (-66.0414, -110.7603) knots 0 0 0 0 1 1 1 1
  spline S1313 degree 3 poles (-66.0414, -110.7603) (-65.9781, -110.6653) (-65.957, -110.6548) (-66.8434, -110.8236) knots 0 0 0 0 1 1 1 1
  spline S1314 degree 3 poles (-58.7183, -111.214) (-58.7183, -111.3301) (-58.6656, -111.3934) (-58.6128, -111.3618) knots 0 0 0 0 1 1 1 1
  spline S1315 degree 3 poles (-58.6128, -111.3618) (-58.5495, -111.3301) (-58.5073, -111.2246) (-58.5073, -111.1402) knots 0 0 0 0 1 1 1 1
  spline S1316 degree 3 poles (-58.5073, -111.1402) (-58.5073, -111.0558) (-58.5495, -110.9925) (-58.6128, -110.9925) knots 0 0 0 0 1 1 1 1
  spline S1317 degree 3 poles (-58.6128, -110.9925) (-58.6656, -110.9925) (-58.7183, -111.0874) (-58.7183, -111.214) knots 0 0 0 0 1 1 1 1
  spline S1318 degree 3 poles (-51.1209, -111.3618) (-51.2053, -111.4567) (-51.2053, -111.5201) (-51.142, -111.5201) knots 0 0 0 0 1 1 1 1
  spline S1319 degree 3 poles (-51.142, -111.5201) (-51.0153, -111.5201) (-50.8676, -111.3196) (-50.9415, -111.2457) knots 0 0 0 0 1 1 1 1
  spline S1320 degree 3 poles (-50.9415, -111.2457) (-50.9626, -111.2246) (-51.047, -111.2668) (-51.1209, -111.3618) knots 0 0 0 0 1 1 1 1
  spline S1321 degree 3 poles (-45.37, -111.404) (-45.4966, -111.4567) (-45.2645, -111.5095) (-44.6841, -111.5517) knots 0 0 0 0 1 1 1 1
  spline S1322 degree 3 poles (-44.6841, -111.5517) (-44.1882, -111.5834) (-43.6922, -111.6467) (-43.5762, -111.6889) knots 0 0 0 0 1 1 1 1
  spline S1323 degree 3 poles (-43.5762, -111.6889) (-43.4284, -111.7417) (-43.3968, -111.7311) (-43.4706, -111.6467) knots 0 0 0 0 1 1 1 1
  spline S1324 degree 3 poles (-43.4706, -111.6467) (-43.5234, -111.5834) (-43.8083, -111.499) (-44.1038, -111.4673) knots 0 0 0 0 1 1 1 1
  spline S1325 degree 3 poles (-44.1038, -111.4673) (-44.3887, -111.4356) (-44.7474, -111.3829) (-44.8952, -111.3618) knots 0 0 0 0 1 1 1 1
  spline S1326 degree 3 poles (-44.8952, -111.3618) (-45.0429, -111.3407) (-45.2539, -111.3618) (-45.37, -111.404) knots 0 0 0 0 1 1 1 1
  spline S1327 degree 3 poles (-69.0065, -114.8123) (-69.6502, -115.361) (-70.7371, -116.469) (-71.2858, -117.1443) knots 0 0 0 0 1 1 1 1